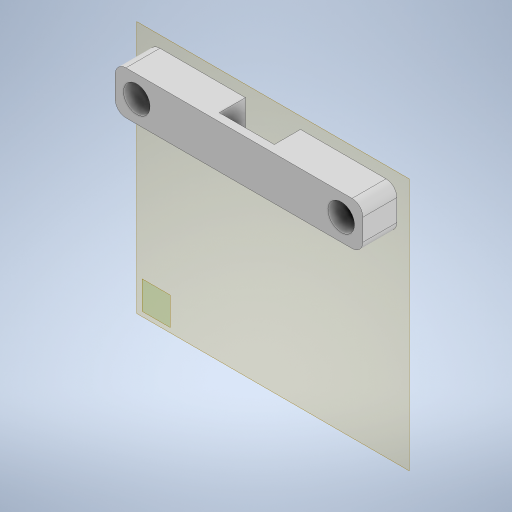
# Autodesk Inventor part: connectorHolder_V6
Saved by Autodesk Inventor 2023 (Build 270158000, 158)
## iProperties
Created: 2023-03-19
Part Number: connectorHolder_V6
Material: Generic
Document SubType Name: Modeling
Designer: shrey
Density: 1 g/cm^3
Appearance: Default
Author: shrey
Autodesk Inventor part; units mm, degrees
ref_plane "YZ Plane" through (0, 0, 0) normal (1, 0, 0) x (0, 1, 0)
ref_plane "XZ Plane" through (0, 0, 0) normal (0, 1, 0) x (-1, 0, 0)
ref_plane "XY Plane" through (0, 0, 0) normal (0, 0, 1) x (1, 0, 0)
ref_plane "Work Plane1" through (-28.594, 4.5215, 39.249) normal (0, 0, 1) x (1, 0, 0)
sketch "Sketch1" plane through (-28.594, 4.5215, 39.249) normal (0, 0, 1) x (1, 0, 0)
  circle A0 centre (23.594, 21.5215) radius 1.45 projected
  circle A1 centre (-23.594, 21.5215) radius 1.45 projected
  circle A2 centre (23.594, 21.5215) radius 1.45 projected
  arc A3 (-26.094, 26.5215) -> (-28.594, 24.0215) centre (-26.094, 24.0215) ccw projected
  line L0 (26.094, 26.5215) -> (-26.094, 26.5215) projected
  arc A4 (28.594, 24.0215) -> (26.094, 26.5215) centre (26.094, 24.0215) ccw projected
  line L1 (28.594, 19.0215) -> (28.594, 24.0215) projected
  arc A5 (26.094, 16.5215) -> (28.594, 19.0215) centre (26.094, 19.0215) ccw projected
  line L2 (-26.094, 16.5215) -> (26.094, 16.5215) projected
  arc A6 (-28.594, 19.0215) -> (-26.094, 16.5215) centre (-26.094, 19.0215) ccw projected
  line L3 (-28.594, 24.0215) -> (-28.594, 19.0215) projected
  circle A7 centre (-23.594, 21.5215) radius 1.45 projected
  point P0 (28.594, -4.5215)
extrude "Extrusion1" add sketch "Sketch1" along normal blind 7.842
sketch "Sketch2" plane through (-54.688, 31.043, 39.249) normal (0, 1, 0) x (1, 0, 0)
  line L0 (32.3438, -5.842) -> (19.8438, -5.842) construction
  line L1 (19.8438, -5.842) -> (19.8438, 0) construction
  line L2 (19.8438, 0) -> (32.3438, 0) construction
  line L3 (32.3438, 0) -> (32.3438, -5.842) construction
  line L4 (52.188, 0) -> (0, 0) projected
  line L5 (32.4438, 0) -> (32.4438, -6.042)
  line L6 (32.4438, -6.042) -> (19.7438, -6.042)
  line L7 (19.7438, -6.042) -> (19.7438, 0)
  point P0 (54.688, 39.249)
  dimension "d2" = 0.1
  dimension "d3" = 0.1
  dimension "d4" = 0.2
  constraints: 14 end point, 3 perpendicular, 2 parallel, 2 point on line, 1 horizontal, 1 vertical, 2 other
  measures "d2" distance between parallel lines of L7 L1
  measures "d3" distance between parallel lines of L3 L5
  measures "d4" distance between parallel lines of L0 L6
extrude "Extrusion2" cut sketch "Sketch2" against normal blind 12.908
ref_plane "Work Plane2" through (-52.188, -17, 42.6) normal (0, 0, -1) x (0, 1, 0)
sketch "Sketch3" plane through (-52.188, -17, 42.6) normal (0, 0, -1) x (0, 1, 0)
  line L0 (45.543, -5) -> (40.543, -5) projected
  arc A0 (38.043, -2.5) -> (40.543, -5) centre (40.543, -2.5) ccw projected
  line L1 (38.043, -2.5) -> (38.043, 49.688) projected
  arc A1 (40.543, 52.188) -> (38.043, 49.688) centre (40.543, 49.688) ccw projected
  line L2 (40.543, 52.188) -> (45.543, 52.188) projected
  arc A2 (48.043, 49.688) -> (45.543, 52.188) centre (45.543, 49.688) ccw projected
  line L3 (48.043, 49.688) -> (48.043, -2.5) projected
  arc A3 (45.543, -5) -> (48.043, -2.5) centre (45.543, -2.5) ccw projected
  circle A4 centre (43.043, 47.188) radius 1.45 projected
  circle A5 centre (43.043, 0) radius 1.45 projected
  circle A6 centre (0, 47.188) radius 3.065 projected
  circle A7 centre (43.043, 47.188) radius 3.065 projected
  circle A8 centre (43.043, 0) radius 3.065 projected
  point P0 (17, 52.188)
extrude "Extrusion3" cut sketch "Sketch3" against normal blind 12.908 contours A4 | A5 | A7 | A8
body "Solid1"
